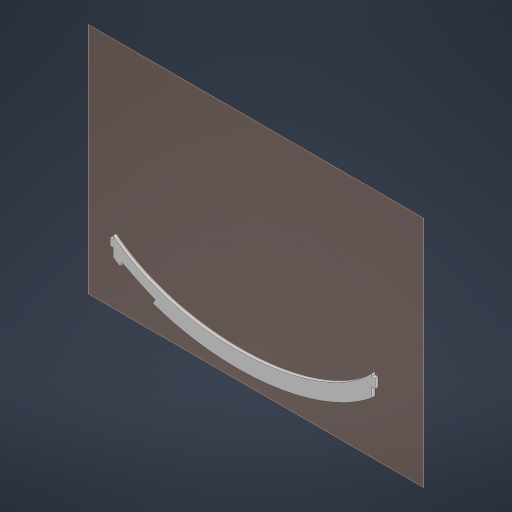
# Autodesk Inventor part: Spant2
Saved by Autodesk Inventor 2023 (Build 270158000, 158)
## iProperties
Created: 2022-06-17
Part Number: Spant2
Material: Generic
Document SubType Name: Modeling
Designer: bananenbrot
Density: 1 g/cm^3
Appearance: Default
Author: bananenbrot
Autodesk Inventor part; units mm, degrees
ref_plane "YZ Plane" through (0, 0, 0) normal (1, 0, 0) x (0, 1, 0)
ref_plane "XZ Plane" through (0, 0, 0) normal (0, 1, 0) x (-1, 0, 0)
ref_plane "XY Plane" through (0, 0, 0) normal (0, 0, 1) x (1, 0, 0)
ref_plane "Work Plane1" through (0, 0, 0) normal (0, 0, 1) x (-1, 0, 0)
sketch "Sketch1" plane through (0, 0, 0) normal (0, 0, 1) x (-1, 0, 0)
  spline S0 degree 3 poles (105.4883, 71.0587) (105.6559, 71.4694) (105.824, 71.88) (106.1569, 72.6904) (106.3216, 73.0904) (106.4867, 73.4901) knots -0.266162 -0.266162 -0.266162 -0.266162 -0.133087 -0.133087 -0.003341 -0.003341 -0.003341 -0.003341
  spline S1 degree 3 poles (106.4867, 73.4901) (99.3414, 77.5054) (91.623, 81.1106) (83.426, 84.2596) knots -25.895552 -25.895552 -25.895552 -25.895552 -23.89596 -23.89596 -23.89596 -23.89596
  spline S2 degree 3 poles (83.426, 84.2596) (83.383, 84.1862) (83.3401, 84.1127) (83.2498, 83.9584) (83.2025, 83.8776) (83.1552, 83.7967) knots -0.053633 -0.053633 -0.053633 -0.053633 -0.028107 -0.028107 0 0 0 0
  spline S3 degree 3 poles (83.1552, 83.7967) (82.995, 83.5034) (82.8346, 83.2101) (82.5137, 82.6238) (82.353, 82.3306) (82.1922, 82.0376) knots -0.200537 -0.200537 -0.200537 -0.200537 -0.100278 -0.100278 -0.000001 -0.000001 -0.000001 -0.000001
  spline S4 degree 3 poles (82.1922, 82.0376) (86.075, 80.3865) (89.9435, 78.6654) (97.7089, 75.0245) (101.6317, 73.0864) (105.4883, 71.0587) knots -2.573015 -2.573015 -2.573015 -2.573015 -1.307167 -1.307167 -0.00005 -0.00005 -0.00005 -0.00005
  spline S5 degree 3 poles (-58.9228, -91.9417) (-58.7749, -91.5277) (-58.6267, -91.1139) (-58.3286, -90.2835) (-58.1787, -89.8669) (-58.0284, -89.4505) knots -0.264733 -0.264733 -0.264733 -0.264733 -0.132868 -0.132868 -0.000055 -0.000055 -0.000055 -0.000055
  spline S6 degree 3 poles (-58.0284, -89.4505) (-62.2238, -88.2949) (-66.4105, -87.0769) (-74.8294, -84.4769) (-79.0836, -83.0842) (-83.2953, -81.6123) knots -2.643421 -2.643421 -2.643421 -2.643421 -1.338468 -1.338468 -0.000018 -0.000018 -0.000018 -0.000018
  spline S7 degree 3 poles (-83.2953, -81.6123) (-83.3681, -81.9392) (-83.4412, -82.2661) (-83.5877, -82.9196) (-83.6612, -83.2462) (-83.7349, -83.5728) knots -0.200918 -0.200918 -0.200918 -0.200918 -0.100445 -0.100445 0 0 0 0
  spline S8 degree 3 poles (-83.7349, -83.5728) (-83.7526, -83.6651) (-83.7703, -83.7574) (-83.8042, -83.9335) (-83.8204, -84.0175) (-83.8365, -84.1014) knots -0.056363 -0.056363 -0.056363 -0.056363 -0.02818 -0.02818 -0.002542 -0.002542 -0.002542 -0.002542
  spline S9 degree 3 poles (-83.8365, -84.1014) (-75.9007, -87.1708) (-67.5641, -89.7922) (-58.9228, -91.9417) knots -18.70759 -18.70759 -18.70759 -18.70759 -16.308401 -16.308401 -16.308401 -16.308401
  spline S10 degree 3 poles (-140.1561, 42.7052) (-140.5265, 42.9467) (-140.897, 43.1882) (-141.6163, 43.6575) (-141.9653, 43.8854) (-142.3142, 44.1132) knots -0.265285 -0.265285 -0.265285 -0.265285 -0.132646 -0.132646 -0.007633 -0.007633 -0.007633 -0.007633
  spline S11 degree 3 poles (-142.3142, 44.1132) (-146.1137, 39.3661) (-149.4383, 34.2577) (-152.1041, 28.8109) knots -4.827939 -4.827939 -4.827939 -4.827939 -3.006582 -3.006582 -3.006582 -3.006582
  spline S12 degree 3 poles (-152.1041, 28.8109) (-152.0643, 28.7818) (-152.0246, 28.7528) (-151.9093, 28.6685) (-151.8337, 28.6133) (-151.7582, 28.5581) knots -0.042842 -0.042842 -0.042842 -0.042842 -0.028073 -0.028073 -0.000004 -0.000004 -0.000004 -0.000004
  spline S13 degree 3 poles (-151.7582, 28.5581) (-151.4839, 28.3673) (-151.2096, 28.1764) (-150.6612, 27.7945) (-150.3869, 27.6033) (-150.1128, 27.4122) knots -0.200499 -0.200499 -0.200499 -0.200499 -0.100262 -0.100262 -0.000004 -0.000004 -0.000004 -0.000004
  spline S14 degree 3 poles (-150.1128, 27.4122) (-148.5536, 30.1288) (-146.8737, 32.8286) (-143.5422, 37.8978) (-141.8646, 40.3248) (-140.1561, 42.7052) knots -1.819993 -1.819993 -1.819993 -1.819993 -0.879034 -0.879034 -0.00001 -0.00001 -0.00001 -0.00001
  spline S15 degree 3 poles (-55.7728, -89.0282) (-55.9385, -89.4734) (-56.1038, -89.9189) (-56.4333, -90.8099) (-56.5976, -91.2556) (-56.7614, -91.7014) knots -0.285003 -0.285003 -0.285003 -0.285003 -0.142483 -0.142483 0 0 0 0
  spline S16 degree 3 poles (-56.7614, -91.7014) (-56.6983, -91.718) (-56.6352, -91.7345) (-56.509, -91.7676) (-56.4459, -91.7842) (-56.3828, -91.8007) knots -0.039143 -0.039143 -0.039143 -0.039143 -0.019569 -0.019569 0 0 0 0
  spline S17 degree 3 poles (-56.3828, -91.8007) (-56.222, -91.32) (-56.0607, -90.8394) (-55.7373, -89.8786) (-55.5752, -89.3983) (-55.4125, -88.9181) knots -0.30413 -0.30413 -0.30413 -0.30413 -0.152078 -0.152078 0 0 0 0
  spline S18 degree 3 poles (-55.4125, -88.9181) (-60.3959, -87.5747) (-65.3718, -86.1432) (-75.3762, -83.0506) (-80.443, -81.3711) (-85.4421, -79.5755) knots -3.141533 -3.141533 -3.141533 -3.141533 -1.593545 -1.593545 0 0 0 0
  spline S19 degree 3 poles (-85.4421, -79.5755) (-85.6008, -80.3472) (-85.7615, -81.1191) (-86.0831, -82.6482) (-86.2442, -83.4064) (-86.4067, -84.1638) knots -0.472496 -0.472496 -0.472496 -0.472496 -0.236135 -0.236135 -0.003733 -0.003733 -0.003733 -0.003733
  spline S20 degree 3 poles (-86.4067, -84.1638) (-90.9201, -82.3538) (-95.299, -80.3975) (-116.0195, -70.1094) (-129.7607, -59.9705) (-146.1593, -41.4596) (-151.3501, -33.6293) (-158.2079, -17.0493) (-159.9962, -8.6553) (-160, -0.0185) (-160, -0.0092) (-160, 0) knots -11.169519 -11.169519 -11.169519 -11.169519 -9.988301 -9.988301 -5.37837 -5.37837 -2.588261 -2.588261 0 0 0.002775 0.002775 0.002775 0.002775
  spline S21 degree 3 poles (-160, 0) (-160, 0.0092) (-160, 0.0185) (-159.9962, 8.6553) (-158.2079, 17.0493) (-154.5318, 25.937) (-154.1376, 26.8372) (-153.7259, 27.7288) knots -31.829362 -31.829362 -31.829362 -31.829362 -31.826146 -31.826146 -28.826161 -28.826161 -28.484445 -28.484445 -28.484445 -28.484445
  spline S22 degree 3 poles (-153.7259, 27.7288) (-153.1336, 27.3124) (-152.5409, 26.8949) (-151.3076, 26.0243) (-150.6649, 25.5695) (-150.024, 25.1147) knots -0.452924 -0.452924 -0.452924 -0.452924 -0.235762 -0.235762 0 0 0 0
  spline S23 degree 3 poles (-150.024, 25.1147) (-148.2187, 28.3868) (-146.2111, 31.6512) (-142.2626, 37.6605) (-140.2732, 40.5119) (-138.2471, 43.2948) knots -2.156978 -2.156978 -2.156978 -2.156978 -1.032693 -1.032693 0 0 0 0
  spline S24 degree 3 poles (-138.2471, 43.2948) (-138.666, 43.5795) (-139.085, 43.8644) (-139.9224, 44.4342) (-140.3412, 44.7193) (-140.7597, 45.0044) knots -0.303868 -0.303868 -0.303868 -0.303868 -0.151928 -0.151928 0 0 0 0
  spline S25 degree 3 poles (-140.7597, 45.0044) (-140.7862, 44.9688) (-140.8126, 44.9333) (-140.8655, 44.8622) (-140.8919, 44.8266) (-140.9183, 44.7911) knots -0.026582 -0.026582 -0.026582 -0.026582 -0.013294 -0.013294 0 0 0 0
  spline S26 degree 3 poles (-140.9183, 44.7911) (-140.5212, 44.5325) (-140.1238, 44.2739) (-139.3291, 43.7572) (-138.9316, 43.4988) (-138.5341, 43.2407) knots -0.284373 -0.284373 -0.284373 -0.284373 -0.142194 -0.142194 0 0 0 0
  spline S27 degree 3 poles (-138.5341, 43.2407) (-140.5827, 40.4214) (-142.5937, 37.5316) (-146.4382, 31.6576) (-148.3257, 28.5856) (-150.0388, 25.5027) knots -2.101071 -2.101071 -2.101071 -2.101071 -1.058051 -1.058051 0 0 0 0
  spline S28 degree 3 poles (-150.0388, 25.5027) (-150.4509, 25.7942) (-150.8636, 26.0856) (-151.6884, 26.6672) (-152.1012, 26.9578) (-152.5139, 27.2479) knots -0.302777 -0.302777 -0.302777 -0.302777 -0.151341 -0.151341 0 0 0 0
  spline S29 degree 3 poles (-152.5139, 27.2479) (-152.7152, 27.3968) (-152.9166, 27.5456) (-153.2728, 27.8086) (-153.4277, 27.9229) (-153.5827, 28.0371) knots -0.150173 -0.150173 -0.150173 -0.150173 -0.075073 -0.075073 -0.017326 -0.017326 -0.017326 -0.017326
  spline S30 degree 3 poles (-153.5827, 28.0371) (-150.1123, 35.463) (-145.4306, 42.2822) (-129.7607, 59.9705) (-116.0195, 70.1094) (-76.1689, 89.896) (-48.1593, 97.1685) (10.3236, 101.4292) (40.3067, 98.6374) (72.6866, 89.1455) (77.3003, 87.6154) (81.772, 85.9536) knots -28.445006 -28.445006 -28.445006 -28.445006 -25.59222 -25.59222 -20.248971 -20.248971 -12.682668 -12.682668 -5.317025 -5.317025 -4.052572 -4.052572 -4.052572 -4.052572
  spline S31 degree 3 poles (81.772, 85.9536) (81.3968, 85.2772) (81.0207, 84.6011) (80.261, 83.24) (79.8771, 82.5546) (79.4924, 81.87) knots -0.467618 -0.467618 -0.467618 -0.467618 -0.235584 -0.235584 0 0 0 0
  spline S32 degree 3 poles (79.4924, 81.87) (84.1061, 79.9441) (88.7048, 77.9202) (97.927, 73.5976) (102.5965, 71.2674) (107.162, 68.806) knots -3.056553 -3.056553 -3.056553 -3.056553 -1.556035 -1.556035 0 0 0 0
  spline S33 degree 3 poles (107.162, 68.806) (107.3625, 69.2729) (107.5637, 69.7398) (107.967, 70.6725) (108.1693, 71.1387) (108.372, 71.6045) knots -0.304859 -0.304859 -0.304859 -0.304859 -0.152403 -0.152403 0 0 0 0
  spline S34 degree 3 poles (108.372, 71.6045) (108.3114, 71.6376) (108.2508, 71.6707) (108.1296, 71.7369) (108.069, 71.7699) (108.0084, 71.8029) knots -0.041431 -0.041431 -0.041431 -0.041431 -0.020705 -0.020705 0 0 0 0
  spline S35 degree 3 poles (108.0084, 71.8029) (107.8317, 71.3605) (107.6555, 70.9178) (107.3043, 70.0319) (107.1293, 69.5884) (106.9549, 69.1449) knots -0.285892 -0.285892 -0.285892 -0.285892 -0.142982 -0.142982 0 0 0 0
  spline S36 degree 3 poles (106.9549, 69.1449) (102.4581, 71.5609) (97.862, 73.8503) (88.8578, 78.0679) (84.4081, 80.0293) (79.9435, 81.8987) knots -2.982662 -2.982662 -2.982662 -2.982662 -1.452066 -1.452066 0 0 0 0
  spline S37 degree 3 poles (79.9435, 81.8987) (80.1899, 82.3388) (80.4359, 82.7793) (80.9269, 83.6602) (81.172, 84.1009) (81.4166, 84.5417) knots -0.302566 -0.302566 -0.302566 -0.302566 -0.151255 -0.151255 0 0 0 0
  spline S38 degree 3 poles (81.4166, 84.5417) (81.5446, 84.757) (81.6725, 84.9724) (81.9225, 85.3939) (82.0446, 85.6002) (82.1667, 85.8065) knots -0.150242 -0.150242 -0.150242 -0.150242 -0.075112 -0.075112 -0.003204 -0.003204 -0.003204 -0.003204
  spline S39 degree 3 poles (82.1667, 85.8065) (96.3401, 80.5048) (109.0798, 73.8828) (120, 66.1438) knots -4.015333 -4.015333 -4.015333 -4.015333 0 0 0 0
  line L0 (120, 66.1438) -> (120, 64.9158)
  spline S40 degree 3 poles (120, 64.9158) (116.958, 67.0958) (113.7696, 69.1883) (110.4451, 71.1884) knots -27.230162 -27.230162 -27.230162 -27.230162 -26.2705 -26.2705 -26.2705 -26.2705
  spline S41 degree 3 poles (110.4451, 71.1884) (110.1445, 70.4793) (109.8452, 69.769) (109.2415, 68.3271) (108.9366, 67.5943) (108.6339, 66.8613) knots -0.468981 -0.468981 -0.468981 -0.468981 -0.237923 -0.237923 -0.000011 -0.000011 -0.000011 -0.000011
  spline S42 degree 3 poles (108.6339, 66.8613) (103.4133, 69.7415) (98.0406, 72.4439) (87.5696, 77.3439) (82.4064, 79.5941) (77.2296, 81.7217) knots -3.467821 -3.467821 -3.467821 -3.467821 -1.679111 -1.679111 -0.000008 -0.000008 -0.000008 -0.000008
  spline S43 degree 3 poles (77.2296, 81.7217) (77.6144, 82.3927) (77.9981, 83.0647) (78.7561, 84.3968) (79.1306, 85.0574) (79.504, 85.7183) knots -0.463944 -0.463944 -0.463944 -0.463944 -0.231888 -0.231888 -0.004157 -0.004157 -0.004157 -0.004157
  spline S44 degree 3 poles (79.504, 85.7183) (76.0004, 86.9793) (72.415, 88.1586) (41.4117, 97.4273) (11.7123, 100.3449) (-46.585, 96.4605) (-74.7083, 89.3312) (-114.7844, 69.7233) (-128.6069, 59.6354) (-139.3968, 47.5895) (-139.9204, 46.9907) (-140.4363, 46.3856) knots -23.579938 -23.579938 -23.579938 -23.579938 -22.740514 -22.740514 -16.469513 -16.469513 -9.96116 -9.96116 -5.360215 -5.360215 -5.122195 -5.122195 -5.122195 -5.122195
  spline S45 degree 3 poles (-140.4363, 46.3856) (-139.8213, 45.9676) (-139.2057, 45.5495) (-137.9379, 44.6893) (-137.2846, 44.2465) (-136.6316, 43.8045) knots -0.459695 -0.459695 -0.459695 -0.459695 -0.236626 -0.236626 -0.000067 -0.000067 -0.000067 -0.000067
  spline S46 degree 3 poles (-136.6316, 43.8045) (-139.0543, 40.5163) (-141.435, 37.1237) (-145.8862, 30.2958) (-148.0558, 26.7109) (-149.9507, 23.1379) knots -2.432531 -2.432531 -2.432531 -2.432531 -1.213323 -1.213323 -0.000041 -0.000041 -0.000041 -0.000041
  spline S47 degree 3 poles (-149.9507, 23.1379) (-150.5793, 23.5926) (-151.2102, 24.0472) (-152.4036, 24.904) (-152.9683, 25.3083) (-153.5328, 25.7113) knots -0.46512 -0.46512 -0.46512 -0.46512 -0.232385 -0.232385 -0.024389 -0.024389 -0.024389 -0.024389
  spline S48 degree 3 poles (-153.5328, 25.7113) (-153.6538, 25.4318) (-153.773, 25.1514) (-157.1991, 16.9475) (-158.9961, 8.6066) (-159, 0.0184) (-159, 0.0092) (-159, 0) knots -2.665061 -2.665061 -2.665061 -2.665061 -2.573705 -2.573705 0 0 0.002756 0.002756 0.002756 0.002756
  spline S49 degree 3 poles (-159, 0) (-159, -0.0092) (-159, -0.0184) (-158.9961, -8.6066) (-157.1991, -16.9475) (-150.3081, -33.4479) (-145.0794, -41.2454) (-128.6069, -59.6354) (-114.7844, -69.7233) (-94.9296, -79.4376) (-91.5828, -80.947) (-88.1549, -82.3704) knots -31.860137 -31.860137 -31.860137 -31.860137 -31.856914 -31.856914 -28.845903 -28.845903 -25.585929 -25.585929 -20.203225 -20.203225 -19.146895 -19.146895 -19.146895 -19.146895
  spline S50 degree 3 poles (-88.1549, -82.3704) (-88.0052, -81.6256) (-87.8572, -80.88) (-87.5617, -79.3716) (-87.4141, -78.6078) (-87.2687, -77.844) knots -0.461141 -0.461141 -0.461141 -0.461141 -0.233241 -0.233241 -0.000001 -0.000001 -0.000001 -0.000001
  spline S51 degree 3 poles (-87.2687, -77.844) (-81.5487, -79.9485) (-75.7304, -81.8959) (-64.3706, -85.4046) (-58.7727, -86.9978) (-53.1699, -88.4802) knots -3.567329 -3.567329 -3.567329 -3.567329 -1.738656 -1.738656 -0.000005 -0.000005 -0.000005 -0.000005
  spline S52 degree 3 poles (-53.1699, -88.4802) (-53.431, -89.2258) (-53.6908, -89.9722) (-54.2061, -91.4603) (-54.4617, -92.2027) (-54.7161, -92.9452) knots -0.473894 -0.473894 -0.473894 -0.473894 -0.236906 -0.236906 -0.001451 -0.001451 -0.001451 -0.001451
  spline S53 degree 3 poles (-54.7161, -92.9452) (-42.581, -95.7181) (-29.8883, -97.573) (11.7123, -100.3449) (41.4117, -97.4273) (88.331, -83.4004) (105.7686, -75.1143) (120, -64.9158) knots -15.921251 -15.921251 -15.921251 -15.921251 -12.589021 -12.589021 -5.252496 -5.252496 0 0 0 0
  line L1 (120, -64.9158) -> (120, -66.1438)
  spline S54 degree 3 poles (120, -66.1438) (105.5396, -76.3916) (87.8918, -84.6882) (40.3067, -98.6374) (10.3236, -101.4292) (-42.6253, -97.5717) (-65.6494, -92.43) (-85.9727, -84.3372) knots -27.458265 -27.458265 -27.458265 -27.458265 -22.870958 -22.870958 -16.51619 -16.51619 -11.207345 -11.207345 -11.207345 -11.207345
  spline S55 degree 3 poles (-85.9727, -84.3372) (-85.9295, -84.1013) (-85.8864, -83.8654) (-85.7984, -83.3821) (-85.7536, -83.1347) (-85.709, -82.8873) knots -0.147372 -0.147372 -0.147372 -0.147372 -0.075421 -0.075421 0 0 0 0
  spline S56 degree 3 poles (-85.709, -82.8873) (-85.6031, -82.3929) (-85.4977, -81.8982) (-85.2884, -80.9085) (-85.1844, -80.4132) (-85.081, -79.918) knots -0.303476 -0.303476 -0.303476 -0.303476 -0.151784 -0.151784 0 0 0 0
  spline S57 degree 3 poles (-85.081, -79.918) (-80.1681, -81.6744) (-75.1908, -83.3195) (-65.4257, -86.3336) (-60.6031, -87.7222) (-55.7728, -89.0282) knots -3.066818 -3.066818 -3.066818 -3.066818 -1.501137 -1.501137 0 0 0 0
  line L2 (-130, 8.1062) -> (-130, 56.9656) projected
  line L3 (-130, 56.9656) -> (-130, 45.8815)
  line L4 (120, 64.9158) -> (120, 46.4329)
  ellipse E0 centre (0, 0) end of major axis (0, 84.0004) minor radius 144
  line L5 (-217.5271, 0) -> (185.1628, 0)
  line L6 (0, -140) -> (0, 140)
  point P0 (-144, 0)
  point P1 (0, 99.0004)
  point P2 (0, 84.0004)
  point P3 (-130, 36.1292)
  dimension "d0" = 15
  dimension "d1" = 15
  constraints: 12 end point, 4 point on line, 4 vertical, 1 coincident, 1 horizontal, 240 other
  measures "d0" distance of point (-144, 0) point (-159, 0)
  measures "d1" distance of point (0, 99) point (0, 84)
extrude "Extrusion1" add sketch "Sketch1" along normal mid plane 3 contours L2 S44 L6 E0 | E0 L6 S44 S43 S42 S41 S40 L4
sketch "Sketch2" plane through (0, 0, 1.5) normal (0, 0, 1) x (1, 0, 0)
  line L0 (-120, -46.4329) -> (-120, -64.9158) projected
  line L1 (130, -56.9656) -> (130, -36.1292) projected
  line L2 (130, -42.1292) -> (127, -42.1292)
  line L3 (127, -42.1292) -> (127, -31.2453)
  line L4 (127, -31.2453) -> (130, -31.2453)
  line L5 (130, -31.2453) -> (130, -42.1292)
  line L6 (130, -50.9656) -> (127, -50.9656)
  line L7 (127, -50.9656) -> (127, -61.0476)
  line L8 (127, -61.0476) -> (130, -61.0476)
  line L9 (130, -61.0476) -> (130, -50.9656)
  line L10 (-120, -52.4329) -> (-117, -52.4329)
  line L11 (-117, -52.4329) -> (-117, -43.0285)
  line L12 (-117, -43.0285) -> (-120, -43.0285)
  line L13 (-120, -43.0285) -> (-120, -52.4329)
  line L14 (-120, -58.9158) -> (-117, -58.9158)
  line L15 (-117, -58.9158) -> (-117, -71.4096)
  line L16 (-117, -71.4096) -> (-120, -71.4096)
  line L17 (-120, -71.4096) -> (-120, -58.9158)
  point P0 (0, 0)
  point P1 (128.5, -42.1292)
  point P2 (-118.5, -52.4329)
  point P3 (130, -50.9656)
  point P4 (130, -42.1292)
  dimension "d5" = 3
  dimension "d6" = 3
  dimension "d7" = 6
  dimension "d8" = 6
  dimension "d9" = 3
  dimension "d10" = 3
  dimension "d11" = 6
  dimension "d12" = 6
  constraints: 32 end point, 8 parallel, 4 horizontal, 4 perpendicular, 4 point on line, 2 midpoint
  measures "d5" distance of L3.end L4.end
  measures "d6" distance of L8.end L7.end
  measures "d7" vertical distance of L1.end point (128.5, -42.129)
  measures "d8" distance from line of L1.start L6
  measures "d9" distance of L12.end L11.end
  measures "d10" distance of L15.end L16.end
  measures "d11" vertical distance of L0.start point (-118.5, -52.433)
  measures "d12" distance from line of L14 L0.end
extrude "Extrusion2" cut sketch "Sketch2" against normal blind 10
body "Solid1"
